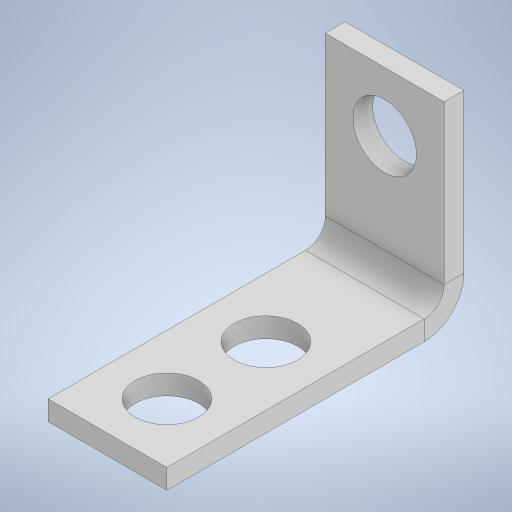
# Autodesk Inventor part: connector2_cooler
Saved by Autodesk Inventor 2023 (Build 270158000, 158)
## iProperties
Created: 2023-06-13
Part Number: connector2_cooler
Material: 一般
Document SubType Name: Sheet Metal
Designer: 310611102
Density: 1 g/cm^3
Sheet Metal Rule: Default_mm
Appearance: 預設
Author: 310611102
Autodesk Inventor part; units mm, degrees
ref_plane "YZ Plane" through (0, 0, 0) normal (1, 0, 0) x (0, 1, 0)
ref_plane "XZ Plane" through (0, 0, 0) normal (0, 1, 0) x (-1, 0, 0)
ref_plane "XY Plane" through (0, 0, 0) normal (0, 0, 1) x (1, 0, 0)
sketch "Sketch1" plane through (0, 0, 0) normal (0, 0, 1) x (1, 0, 0)
  line L0 (-3, 5) -> (3, 5)
  line L1 (3, 5) -> (3, -5)
  line L2 (3, -5) -> (-3, -5)
  line L3 (-3, -5) -> (-3, 5)
  line L4 (-3, 5) -> (3, -5) construction
  line L5 (3, 5) -> (-3, -5) construction
  circle A0 centre (0, 2) radius 1.6
  point P0 (0, 0)
  dimension "d0" = 10
  dimension "d1" = 6
  dimension "d3" = 3.2
  dimension "d4" = 3
  measures "d0" distance of L0.end L1.end
  measures "d1" distance of L0.start L0.end
  measures "d3" diameter of A0
  measures "d4" distance from line of L0 A0.centre
extrude "Plate1" add sketch "Sketch1" along normal blind 1
sketch "Sketch2" plane through (3, -4, 0) normal (0, -1, 0) x (1, 0, 0)
  line L0 (-6, 0) -> (0, 0)
  line L1 (0, 0) -> (0, 15)
  line L2 (0, 15) -> (-6, 15)
  line L3 (-6, 15) -> (-6, 0)
  constraints: 6 end point, 1 horizontal, 1 perpendicular, 1 vertical
edge flange "Flange1" height 15 angle 90 thickness 1 bend radius 1 thickness toward (0, -1, 0) relief tear relief width 1 relief depth 0.5 edges at (0, -5, 1) wall of the first edge with corners at (-3, -4, 0) (3, -4, 0) (3, -4, 15) (-3, -4, 15)
bend "Bend1"
corner "Corner1"
sketch "Sketch3" plane through (-3, -4, 15) normal (0, 1, 0) x (1, 0, 0)
  circle A0 centre (3, 3) radius 1.6
  circle A1 centre (3, 8) radius 1.6
  line L0 (0, 0) -> (6, 0) projected
  point P0 (3, 15)
  point P1 (3, 0)
  dimension "d15" = 3.2
  dimension "d16" = 3.2
  dimension "d17" = 5
  dimension "d18" = 3
  constraints: 2 centre point, 2 vertical alignment, 1 midpoint
  measures "d15" diameter of A0
  measures "d16" diameter of A1
  measures "d17" distance of A1.centre A0.centre
  measures "d18" distance from line of L0 A0.centre
extrude "Cut1" cut sketch "Sketch3" against normal blind 1
equation "\"d19\" = 厚度"
equation "\"d2\" = 厚度"
equation "\"d5\" = 折彎離隙寬度"
equation "\"d6\" = 折彎離隙深度"
equation "\"d7\" = 最小剩餘"
equation "\"d8\" = 轉移半徑"
equation "\"d11\" = 折彎半徑"
equation "\"d12\" = 轉角離隙大小"
equation "\"d13\" = 間隙大小"
equation "\"d14\" = Jacobi半徑大小"
equation "\"折彎半徑\" = 厚度"
equation "\"折彎離隙寬度\" = 厚度"
equation "\"折彎離隙深度\" = 0.5 * 厚度"
equation "\"轉角離隙大小\" = 4 * 厚度"
equation "\"最小剩餘\" = 2 * 厚度"
equation "\"轉移半徑\" = 折彎半徑"
equation "\"Jacobi半徑大小\" = 折彎半徑"
equation "\"間隙大小\" = 厚度"
equation "\"厚度\" = 1"
body "Solid1"
